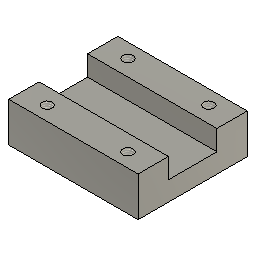
7c811ac5-ca6c-42b8-af26-bc77b9e3022a (Autodesk Fusion 360 design; units mm, degrees)
Autodesk Fusion 360 part; units mm, degrees
sketch "Sketch1" plane through (0, 0, 0) normal (0, 0, 1) x (1, 0, 0)
  line L0 (0, 0) -> (32, 0)
  line L1 (32, 0) -> (32, 27)
  line L2 (32, 27) -> (0, 27)
  line L3 (0, 27) -> (0, 0)
  dimension "d1" = 27
  dimension "d2" = 32
  constraint horizontal L0
  constraint vertical L1
  constraint horizontal L2
  constraint vertical L3
  constraint coincident L0.start L3.end
  measures "d1" distance of L0.start L2.end
  measures "d2" distance of L1.end L2.end
extrude "Extrude1" add sketch "Sketch1" along normal blind 4.8
sketch "Sketch2" plane through (0, 0, 4.8) normal (0, 0, 1) x (-1, 0, 0)
  line L0 (0, -27) -> (0, 0)
  line L1 (0, 0) -> (-32, 0)
  line L2 (-32, 0) -> (-32, -27)
  line L3 (-32, -27) -> (0, -27)
  line L4 (0, 0) -> (-32, 0)
  line L5 (-32, 0) -> (-32, -7.5)
  line L6 (-32, -7.5) -> (0, -7.5)
  line L7 (0, -7.5) -> (0, 0)
  line L8 (-32, -27) -> (0, -27)
  line L9 (0, -27) -> (0, -19.5)
  line L10 (0, -19.5) -> (-32, -19.5)
  line L11 (-32, -19.5) -> (-32, -27)
  dimension "d5" = 12
  dimension "d6" = 7.5
  dimension "d7" = 8.2363
  constraint horizontal L4
  constraint vertical L5
  constraint horizontal L6
  constraint vertical L7
  constraint coincident L2 L5.end
  constraint coincident L0.end L1.start
  constraint horizontal L8
  constraint vertical L9
  constraint horizontal L10
  constraint vertical L11
  constraint coincident L0 L9.end
  constraint coincident L2.end L3.start
  measures "d5" distance of L6 L10
  measures "d6" distance of L0.end L6.end
extrude "Extrude2" add sketch "Sketch2" along normal blind 5 contours L0 L2 L3 L8 L9 L10 L11 | L0 L1 L2 L4 L5 L6 L7
sketch "Sketch3" plane through (0, 0, 0) normal (0, 0, -1) x (1, 0, 0)
  line L0 (0, 0) -> (0, -27)
  line L1 (0, -27) -> (32, -27)
  line L2 (32, -27) -> (32, 0)
  line L3 (32, 0) -> (0, 0)
  line L4 (6, -3.5) -> (26, -3.5)
  line L5 (26, -3.5) -> (26, -23.5)
  line L6 (26, -23.5) -> (6, -23.5)
  line L7 (6, -23.5) -> (6, -3.5)
  circle A0 centre (6, -3.5) radius 1.5
  circle A1 centre (26, -3.5) radius 1.5
  circle A2 centre (6, -23.5) radius 1.5
  circle A3 centre (26, -23.5) radius 1.5
  dimension "d10" = 20
  dimension "d11" = 20
  dimension "d12" = 3.5
  dimension "d13" = 3
  dimension "d14" = 6
  dimension "d15" = 6
  dimension "d16" = 3
  dimension "d17" = 3
  dimension "d18" = 3
  dimension "d19" = 3
  constraint horizontal L4
  constraint vertical L5
  constraint horizontal L6
  constraint vertical L7
  constraint coincident L4.start L7.end
  constraint coincident L4.end L5.start
  constraint coincident L6.end L7.start
  constraint coincident L5.end L6.start
  measures "d10" distance of L4.start L4.end
  measures "d11" distance of L4.end L5.end
  measures "d12" distance of L2.end L4
  measures "d14" horizontal distance of L0.start L4.start
  measures "d15" horizontal distance of L2.end L4.end
  measures "d16" diameter of A0
  measures "d17" diameter of A1
  measures "d18" diameter of A2
  measures "d19" diameter of A3
extrude "Extrude3" cut sketch "Sketch3" against normal blind 20 contours L4 L7 A0 | L4 L7 A0 | L4 L5 A1 | L4 L5 A1 | L6 L7 A2 | L6 L7 A2 | L5 L6 A3 | L5 L6 A3
chamfer "Chamfer1" distance 0.25 angle 45 4 edges at (4.6015, 2.9576, 0) (24.6015, 2.9576, 0) (24.6015, 22.9576, 0) (4.6015, 22.9576, 0)
thread "Thread1" "ISO Metric profile 3.0 M3x0.5 6H" major diameter 3.086 minor diameter 2.529 pitch 0.5 angle 60 resizes the face on face at (7.4925, 23.3506, 3.4333) on face at (27.4925, 23.3506, 3.4333) on face at (27.4981, 3.5748, 6.6167) on face at (7.4981, 3.5748, 6.6167)
